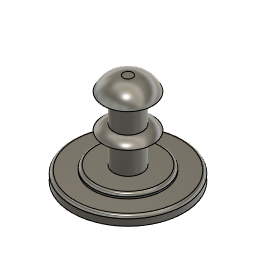
xiaomiButton v4 (Autodesk Fusion 360 design; units mm, degrees)
Autodesk Fusion 360 part; units mm, degrees
note: some values were not read from the file. Set by a fixed rule: which face or edge a step refers to.
sketch "Sketch1" plane through (0, 0, 0) normal (0, 1, 0) x (1, 0, 0)
  circle A0 centre (0, 0) radius 4
  circle A1 centre (0, 0) radius 2.5
  dimension "d1" = 8
  dimension "d2" = 5
  constraint coincident A0.centre A1.centre
  measures "d1" diameter of A0
  measures "d2" diameter of A1
extrude "Extrude1" add sketch "Sketch1" along normal blind 0.8 contours A0 | A1
extrude "Extrude2" add sketch "Sketch1" along normal blind 1.125 contours A1
sketch "Sketch3" plane through (0, 1.125, 0) normal (0, 1, 0) x (-1, 0, 0)
  circle A0 centre (0, 0) radius 2.5
  circle A1 centre (0, 0) radius 1
  dimension "d7" = 2
  constraint coincident A0.centre A1.centre
  measures "d7" diameter of A1
extrude "Extrude3" add sketch "Sketch3" along normal blind 4.5 contours A1
ref_plane "WorkPlane1" through (0, 3.25, 0) normal (0, 1, 0) x (1, 0, 0)
sketch "Sketch4" plane through (0, 3.25, 0) normal (0, 1, 0) x (1, 0, 0)
  circle A0 centre (0, 0) radius 1.75
  dimension "d11" = 3.5
  constraint coincident A0.centre origin
  measures "d11" diameter of A0
extrude "Extrude4" add sketch "Sketch4" along normal blind 0.4
fillet "Fillet1" radius 1 1 edges at (-1.6316, 3.65, 0.6328)
sketch "Sketch5" plane through (0, 5.625, 0) normal (0, 1, 0) x (-1, 0, 0)
  circle A0 centre (0, 0) radius 1
  circle A1 centre (0, 0) radius 1.75
  dimension "d16" = 3.5
  constraint coincident A0.centre A1.centre
  measures "d16" diameter of A1
extrude "Extrude5" add sketch "Sketch5" along normal blind 1 contours A0 | A1
fillet "Fillet2" radius 1.5 1 edges at (1.6316, 6.625, -0.6328)
fillet "Fillet3" radius 0.2 1 edges at (-3.7293, 0.8, 1.4465)
fillet "Fillet4" radius 0.2 1 edges at (-2.3308, 1.125, 0.904)
move_face "OffsetFaces1" offset -0.05 1 faces at (3.995, 0.4, 0.1994)
move_face "OffsetFaces2" offset -0.15 1 faces at (-0.481, 0, -1.2257)
